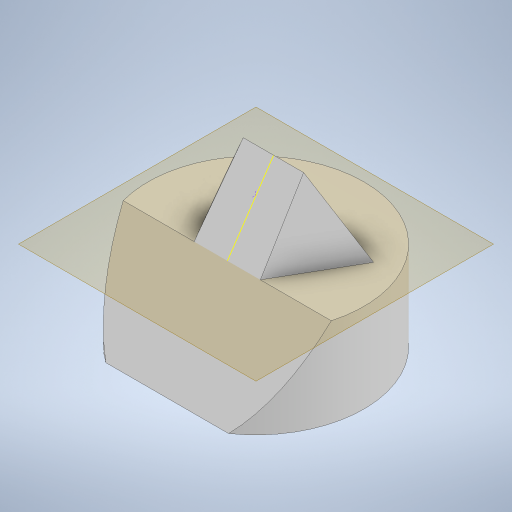
# Autodesk Inventor part: Даник
Saved by Autodesk Inventor 2024 (Build 280153000, 153)
## iProperties
Created: 2023-11-25
Part Number: Даник
Material: Типовые
Document SubType Name: Modeling
Designer: User
Density: 1 g/cm^3
Appearance: По умолчанию
Author: User
Autodesk Inventor part; units mm, degrees
ref_plane "YZ Plane" through (0, 0, 0) normal (1, 0, 0) x (0, 1, 0)
ref_plane "XZ Plane" through (0, 0, 0) normal (0, 1, 0) x (-1, 0, 0)
ref_plane "XY Plane" through (0, 0, 0) normal (0, 0, 1) x (1, 0, 0)
sketch "Эскиз1" plane through (0, 0, 0) normal (0, 1, 0) x (-1, 0, 0)
  circle A0 centre (0, 0) radius 30.3329
  constraints: 1 centre point, 1 coincident
extrude "Выдавливание1" add sketch "Эскиз1" along normal blind 25
sketch "Эскиз2" plane through (0, 25, 0) normal (0, 1, 0) x (1, 0, 0)
  circle A0 centre (0, 0) radius 24.1972
  line L0 (0, -24.1972) -> (-20.9554, 12.0986)
  line L1 (-20.9554, 12.0986) -> (20.9554, 12.0986)
  line L2 (20.9554, 12.0986) -> (0, -24.1972)
  constraints: 6 end point, 2 coincident, 1 vertical alignment, 9 other
ref_plane "РабПлоскость1" through (0, 25, 0) normal (0, 1, 0) x (1, 0, 0)
sketch "Эскиз3" plane through (0, 0, 0) normal (1, 0, 0) x (0, 1, 0)
  point P0 (0, 0)
  point P1 (57.2818, 0)
loft "Лофт1" add profiles "Эскиз2" section 1 point at (0, 57.2818, 0) contours L2 L0 L1
sketch "Эскиз4" plane through (0, 0, 0) normal (1, 0, 0) x (0, 1, 0)
  line L0 (57.2818, 0) -> (25, -12.0986) projected
  line L1 (44.209, -4.8994) -> (0, 24.9536)
  line L2 (0, -30.3329) -> (0, 30.3329) projected
  line L3 (44.209, -4.8994) -> (65.2796, 2.9974)
  line L4 (65.2796, 2.9974) -> (0, 50.3359)
  line L5 (0, 50.3359) -> (0, 24.9536)
  point P0 (0, 0)
  constraints: 8 end point, 2 point on line, 1 vertical
extrude "Выдавливание2" cut sketch "Эскиз4" along normal blind 356 and the other way blind 435
sketch "Эскиз5" plane through (0, 0, 0) normal (1, 0, 0) x (0, 1, 0)
  line L0 (25, 8.0718) -> (44.209, -4.8994) projected
  point P0 (0, 0)
  point P1 (36.9535, 0)
  constraints: 1 point on line
